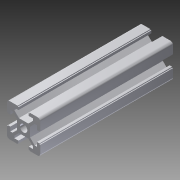
# Autodesk Inventor part: 20x20 Slotted Extrusion Stationary Arm
Saved by Autodesk Inventor 2015 SP1 (Build 190203100, 203)
## iProperties
Created: 2015-03-03
Part Number: 20x20 Slotted Extrusion Stationary Arm
Material: Aluminum 6061
Document SubType Name: Modeling
Designer: Andrew
Density: 2.7 g/cm^3
Appearance: Aluminum - Flat
Author: Andrew
Autodesk Inventor part; units mm, degrees
ref_plane "YZ Plane" through (0, 0, 0) normal (1, 0, 0) x (0, 1, 0)
ref_plane "XZ Plane" through (0, 0, 0) normal (0, 1, 0) x (-1, 0, 0)
ref_plane "XY Plane" through (0, 0, 0) normal (0, 0, 1) x (1, 0, 0)
sketch "Sketch1" plane through (0, 0, 0) normal (0, 1, 0) x (-1, 0, 0)
  line L0 (10, 10) -> (10, 3.6)
  line L1 (9.5, 3.1) -> (8, 3.1)
  line L2 (8, 3.1) -> (8, 5.63)
  line L3 (8, 5.63) -> (6.6907, 5.63)
  line L4 (6.6907, 5.63) -> (3.9, 2.8393)
  line L5 (2.8393, 3.9) -> (5.63, 6.6907)
  line L6 (5.63, 8) -> (5.63, 6.6907)
  line L7 (5.63, 8) -> (3.1, 8)
  line L8 (3.1, 8) -> (3.1, 9.5)
  line L9 (3.6, 10) -> (10, 10)
  line L10 (-2, 0) -> (12, 0) projected
  line L11 (0, -2) -> (0, 12) projected
  line L12 (3.9, 2.8393) -> (3.9, 0)
  line L13 (2.8393, 3.9) -> (0, 3.9)
  line L14 (0, 0) -> (10, 10) construction
  line L15 (10, 3.6) -> (9.5, 3.6)
  line L16 (9.5, 3.6) -> (9.5, 3.1)
  line L17 (3.6, 10) -> (3.6, 9.5)
  line L18 (3.6, 9.5) -> (3.1, 9.5)
  dimension "d0" = 45
  dimension "d1" = 5.63
  dimension "d2" = 10
  dimension "d3" = 3.1
  dimension "d5" = 6.1
  dimension "d6" = 1.5
  dimension "d7" = 2
  dimension "d11" = 3.6
  constraints: 34 end point, 12 perpendicular, 4 symmetric about line, 2 point on line, 2 vertical, 1 horizontal, 1 parallel, 1 other
  measures "d0" angle of L10 L14
  measures "d1" distance between parallel lines of L10 L3
  measures "d2" distance between parallel lines of L9 L10
  measures "d3" distance between parallel lines of L1 L10
  measures "d5" distance between parallel lines of L12 L0
  measures "d6" distance between parallel lines of L5 L4
  measures "d7" distance between parallel lines of L9 L7
  measures "d11" distance between parallel lines of L10 L15
extrude "Extrusion1" add sketch "Sketch1" along normal mid plane 80
fillet "Fillet1" radius 1.5 1 edges at (-10, 0, 10)
mirror "Mirror1" about plane through (0, 0, 3.9) normal (1, 0, 0)
mirror "Mirror2" about plane through (0, 0, 0) normal (0, 0, -1)
sketch "Sketch2" plane through (0, -40, 0) normal (0, -1, 0) x (1, 0, 0)
  circle A0 centre (0, 0) radius 2.225
  dimension "d12" = 4.45
  constraints: 1 centre point, 1 coincident
  measures "d12" diameter of A0
extrude "Extrusion2" cut sketch "Sketch2" against normal up to next
body "Solid1"
